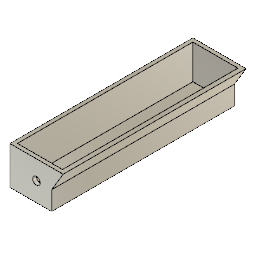
dispenser box tube holder v5 (Autodesk Fusion 360 design; units mm, degrees)
Autodesk Fusion 360 part; units mm, degrees
sketch "side" plane through (0, 0, 0) normal (0, 1, 0) x (1, 0, 0)
  line L0 (0, 0) -> (55, 0)
  line L1 (55, 0) -> (55, -25)
  line L2 (55, -25) -> (70, -50)
  line L3 (70, -50) -> (0, -50)
  line L4 (0, -50) -> (0, 0)
  dimension "d1" = 70
  dimension "d2" = 59.036
  dimension "d3" = 50
  dimension "d4" = 25
  constraint coincident L0.start L4.end
  constraint horizontal L0
  constraint perpendicular L0 L1
  constraint perpendicular L0 L4
  constraint perpendicular L3 L4
  measures "d1" distance of L2.end L3.end
  measures "d2" angle of L2 L3
  measures "d3" distance of L3.end L0.start
  measures "d4" distance of L0.end L1.end
extrude "Extrude1" add sketch "side" along normal blind 240
shell "Shell1" thickness 5 removed faces 1 at (46.6667, 80, 50)
sketch "actuator hole" plane through (0, 0, 0) normal (0, -1, 0) x (1, 0, 0)
  line L0 (70, 50) -> (0, 50)
  line L1 (0, 50) -> (0, 0)
  line L2 (0, 0) -> (55, 0)
  line L3 (55, 0) -> (55, 25)
  line L4 (55, 25) -> (70, 50)
  circle A0 centre (35, 25) radius 5
  line L5 (35, 50) -> (35, 0)
  line L6 (0, 25) -> (15, 25)
  line L7 (15, 25) -> (55, 25)
  dimension "d8" = 10
  constraint midpoint L0 L5.start
  constraint coincident L2 L5.end
  constraint perpendicular L2 L5
  constraint coincident L1 L6.start
  constraint perpendicular L1 L6
  constraint coincident L3.end L4.start
  constraint midpoint L5 L7
  constraint midpoint A0.centre L5
  measures "d8" diameter of A0
extrude "Extrude2" cut sketch "actuator hole" against normal blind 230 contours A0 L5 L7 | A0 L5 L7 | A0 L5 L7 | A0 L5 L7
